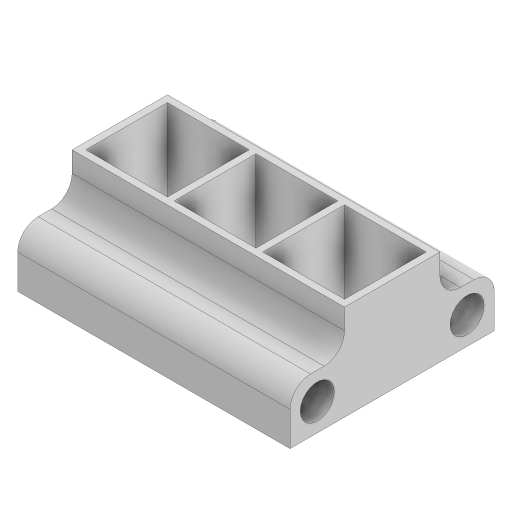
# Autodesk Inventor part: Mould
Saved by Autodesk Inventor 2023 (Build 270158000, 158)
## iProperties
Created: 2026-05-19
Part Number: Mould
Material: Generic
Document SubType Name: Modeling
Designer: ferrerx
Density: 1 g/cm^3
Appearance: Default
Author: ferrerx
Autodesk Inventor part; units mm, degrees
ref_plane "YZ Plane" through (0, 0, 0) normal (1, 0, 0) x (0, 1, 0)
ref_plane "XZ Plane" through (0, 0, 0) normal (0, 1, 0) x (-1, 0, 0)
ref_plane "XY Plane" through (0, 0, 0) normal (0, 0, 1) x (1, 0, 0)
sketch "Sketch1" plane through (0, 0, 0) normal (0, 1, 0) x (-1, 0, 0)
  line L0 (-7, 7) -> (7, 7)
  line L1 (7, 7) -> (7, -7)
  line L2 (7, -7) -> (-7, -7)
  line L3 (-7, -7) -> (-7, 7)
  line L4 (-7, 7) -> (7, -7) construction
  line L5 (7, 7) -> (-7, -7) construction
  point P0 (0, 0)
  dimension "d0" = 14
  dimension "d1" = 14
  constraints: 12 end point, 2 midpoint, 2 parallel, 1 horizontal, 1 perpendicular
  measures "d0" distance of L0.end L1.end
  measures "d1" distance of L1.end L2.end
extrude "Extrusion1" add sketch "Sketch1" along normal blind 14
sketch "Sketch2" plane through (0, 14, 0) normal (0, 1, 0) x (1, 0, 0)
  line L0 (6, -6) -> (-6, -6)
  line L1 (-6, -6) -> (-6, 6)
  line L2 (-6, 6) -> (6, 6)
  line L3 (6, 6) -> (6, -6)
  line L4 (6, -6) -> (-6, 6) construction
  line L5 (-6, -6) -> (6, 6) construction
  point P0 (0, 0)
  dimension "d4" = 12
  dimension "d5" = 12
  constraints: 12 end point, 2 midpoint, 2 parallel, 1 horizontal, 1 perpendicular
  measures "d4" distance of L1.end L2.end
  measures "d5" distance of L0.end L1.end
extrude "Extrusion2" cut sketch "Sketch2" against normal blind 12 draft -2
pattern_linear "Rectangular Pattern1" count 3 spacing 13 along (1, 0, 0) of "Extrusion2", "Extrusion1"
sketch "Sketch3" plane through (33, 0, 7) normal (1, 0, 0) x (0, 0, -1)
  line L0 (0, 0) -> (0, 14) projected
  line L1 (0, 0) -> (-8, 0)
  line L2 (-8, 0) -> (-8, 8)
  line L3 (-8, 8) -> (0, 8)
  line L4 (0, 8) -> (0, 0)
  line L5 (-4, 8) -> (-4, 0) construction
  circle A0 centre (-4, 4) radius 2.5
  point P0 (7, 0)
  dimension "d11" = 8
  dimension "d12" = 8
  dimension "d13" = 5
  constraints: 10 end point, 3 midpoint, 2 parallel, 1 centre point, 1 horizontal, 1 perpendicular
  measures "d11" distance of L2.end L3.end
  measures "d12" distance of L1.end L2.end
  measures "d13" diameter of A0
extrude "Extrusion3" add sketch "Sketch3" against normal up to surface (40 mm away)
fillet "Fillet1" radius 3 2 edges at (13, 8, 15) (13, 8, 7)
mirror "Mirror1" about plane through (0, 0, 0) normal (0, 0, 1) of "Fillet1", "Extrusion3"
fillet_without_effect "Fillet2"
body "Solid1"
